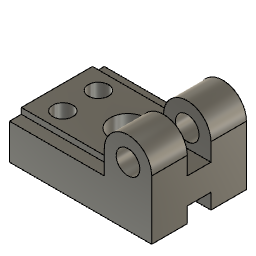
drawing_16 v1 (Autodesk Fusion 360 design; units mm, degrees)
Autodesk Fusion 360 part; units mm, degrees
sketch "Sketch1" plane through (0, 0, 0) normal (0, 0, 1) x (1, 0, 0)
  line L0 (0, 0) -> (-60, 0)
  line L1 (-60, 0) -> (60, 0)
  line L2 (-60, 0) -> (-60, 40)
  line L3 (60, 0) -> (60, -40)
  line L4 (-60, 40) -> (60, 40)
  line L5 (60, 40) -> (60, -40)
  line L6 (60, -40) -> (-60, -40)
  line L7 (-60, -40) -> (-60, 40)
  dimension "d1" = 60
  dimension "d2" = 120
  dimension "d3" = 40
  dimension "d4" = 40
  constraint coincident L0.start origin
  constraint horizontal L0
  constraint parallel L0 L1
  constraint perpendicular L0 L2
  constraint perpendicular L1 L3
  constraint horizontal L4
  constraint vertical L5
  constraint horizontal L6
  constraint vertical L7
  measures "d1" distance of L0.start L0.end
  measures "d2" distance of L0.end L1.end
  measures "d3" distance of L0.end L2.end
  measures "d4" distance of L1.end L3.end
extrude "Extrude1" add sketch "Sketch1" along normal blind 35
sketch "Sketch2" plane through (0, 0, 35) normal (0, 0, 1) x (-1, 0, 0)
  line L0 (60, 40) -> (-60, 40)
  line L1 (-60, 40) -> (-60, -40)
  line L2 (-60, -40) -> (60, -40)
  line L3 (60, -40) -> (60, 40)
  line L4 (-60, -40) -> (40, -40)
  line L5 (60, 0) -> (60, -15)
  line L6 (60, 0) -> (60, 15)
  circle A0 centre (40, -15) radius 8.5
  circle A1 centre (40, 15) radius 8.5
  dimension "d10" = 17
  dimension "d11" = 17
  constraint coincident L1.end L2.start
  constraint perpendicular L1 L4
  constraint midpoint L3 L5.start
  constraint parallel L3 L5
  constraint parallel L3 L6
  measures "d10" diameter of A0
  measures "d11" diameter of A1
extrude "Extrude2" cut sketch "Sketch2" against normal blind 70 contours A0 | A1
sketch "Sketch3" plane through (0, 0, 35) normal (0, 0, 1) x (-1, 0, 0)
  circle A0 centre (40, -15) radius 8.5
  circle A1 centre (40, 15) radius 8.5
  line L0 (60, 40) -> (-60, 40)
  line L1 (-60, 40) -> (-60, -40)
  line L2 (-60, -40) -> (60, -40)
  line L3 (60, -40) -> (60, 40)
  line L4 (-60, 40) -> (0, 40)
  circle A2 centre (0, 0) radius 9
  dimension "d14" = 60
  dimension "d15" = 18
  constraint coincident L0.end L1.start
  constraint perpendicular L1 L4
  constraint coincident A2.centre origin
  measures "d14" distance of L0.end L4.end
  measures "d15" diameter of A2
extrude "Extrude3" cut sketch "Sketch3" against normal blind 55 contours A2
sketch "Sketch4" plane through (0, 0, 35) normal (0, 0, 1) x (-1, 0, 0)
  circle A0 centre (0, 0) radius 9
  circle A1 centre (40, -15) radius 8.5
  circle A2 centre (40, 15) radius 8.5
  line L0 (60, 40) -> (-60, 40)
  line L1 (-60, 40) -> (-60, -40)
  line L2 (-60, -40) -> (60, -40)
  line L3 (60, -40) -> (60, 40)
  circle A3 centre (0, 0) radius 15
  dimension "d18" = 30
  constraint coincident A0.centre A3.centre
  measures "d18" diameter of A3
extrude "Extrude4" cut sketch "Sketch4" against normal blind 17 contours A3
sketch "Sketch5" plane through (0, 40, 0) normal (0, 1, 0) x (-1, 0, 0)
  line L0 (-60, 0) -> (60, 0)
  line L1 (60, 0) -> (60, 35)
  line L2 (60, 35) -> (-60, 35)
  line L3 (-60, 35) -> (-60, 0)
  line L4 (-60, 0) -> (-40, 0)
  line L5 (-60, 0) -> (-60, 50)
  line L6 (-20, 50) -> (-20, 0)
  arc A0 (-20, 50) -> (-60, 50) centre (-40, 50) ccw
  dimension "d21" = 20
  dimension "d22" = 50
  dimension "d23" = 40
  constraint coincident L0.start L3.end
  constraint perpendicular L3 L4
  constraint tangent L5 A0
  constraint coincident L0 L6.end
  constraint tangent L6 A0
  constraint perpendicular L0 L6
  measures "d21" distance of L0.start L4.end
  measures "d22" distance of L4.end A0.centre
  measures "d23" diameter of A0
extrude "Extrude5" add sketch "Sketch5" against normal blind 80 contours L0 L2 L3 L4 L5 L6 | L2 L5 L6 A0
sketch "Sketch6" plane through (0, 40, 0) normal (0, 1, 0) x (-1, 0, 0)
  line L0 (-60, 0) -> (60, 0)
  line L1 (60, 0) -> (60, 35)
  line L2 (60, 35) -> (-20, 35)
  line L3 (-20, 35) -> (-20, 50)
  arc A0 (-20, 50) -> (-60, 50) centre (-40, 50) ccw
  line L4 (-60, 50) -> (-60, 0)
  circle A1 centre (-40, 50) radius 10
  dimension "d26" = 20
  constraint concentric A0 A1
  measures "d26" diameter of A1
extrude "Extrude6" cut sketch "Sketch6" against normal blind 95 contours A1
sketch "Sketch7" plane through (0, 0, 35) normal (0, 0, 1) x (-1, 0, 0)
  line L0 (-20, 40) -> (-20, -40)
  line L1 (-20, -40) -> (60, -40)
  line L2 (60, -40) -> (60, 40)
  line L3 (60, 40) -> (-20, 40)
  circle A0 centre (0, 0) radius 15
  circle A1 centre (40, -15) radius 8.5
  circle A2 centre (40, 15) radius 8.5
  line L4 (60, 40) -> (60, 30) construction
  line L5 (60, -40) -> (60, -30) construction
  line L6 (60, -40) -> (-20, -40)
  line L7 (-20, -40) -> (-20, -30)
  line L8 (-20, -30) -> (60, -30)
  line L9 (60, -30) -> (60, -40)
  line L10 (60, 30) -> (-20, 30)
  line L11 (-20, 30) -> (-20, 40)
  line L12 (-20, 40) -> (60, 40)
  line L13 (60, 40) -> (60, 30)
  constraint coincident L2.end L3.start
  constraint perpendicular L3 L4
  constraint coincident L1.end L2.start
  constraint coincident L2 L5.end
  constraint perpendicular L1 L5
  constraint horizontal L6
  constraint vertical L7
  constraint horizontal L8
  constraint vertical L9
  constraint coincident L0 L7.end
  constraint horizontal L10
  constraint vertical L11
  constraint horizontal L12
  constraint vertical L13
  constraint coincident L0.start L3.end
extrude "Extrude7" cut sketch "Sketch7" against normal blind 5 contours L0 L2 L3 L10 L11 L12 L13 | L0 L1 L2 L6 L7 L8 L9
ref_plane "WorkPlane1" through (0, 0, 35) normal (0, 0, 1) x (1, 0, 0)
sketch "Sketch8" plane through (0, 0, 35) normal (0, 0, 1) x (1, 0, 0)
  line L0 (60, -40) -> (-60, -40)
  line L1 (-60, -40) -> (-60, 40)
  line L2 (-60, 40) -> (60, 40)
  line L3 (60, 40) -> (60, -40)
  circle A0 centre (-40, -15) radius 8.5
  circle A1 centre (-40, 15) radius 8.5
  circle A2 centre (0, 0) radius 9
  line L4 (60, 0) -> (30, 0) construction
  line L5 (30, 0) -> (20, 0) construction
  line L6 (20, 0) -> (20, 10) construction
  line L7 (20, 10) -> (20, -10)
  line L8 (20, -10) -> (67.6256, -10)
  line L9 (67.6256, -10) -> (67.6256, 10)
  line L10 (67.6256, 10) -> (20, 10)
  dimension "d33" = 30
  dimension "d34" = 10
  dimension "d35" = 20
  constraint horizontal L4
  constraint parallel L4 L5
  constraint perpendicular L5 L6
  constraint perpendicular L5 L7
  constraint perpendicular L3 L8
  constraint perpendicular L8 L9
  constraint perpendicular L7 L10
  measures "d33" distance of L4.start L4.end
  measures "d34" distance of L5.end L6.end
  measures "d35" distance of L6.end L7.end
extrude "Extrude8" cut sketch "Sketch8" along normal blind 90 contours L3 L7 L8 L10 | L3 L8 L9 L10
sketch "Sketch9" plane through (0, 0, 0) normal (0, 0, -1) x (1, 0, 0)
  line L0 (60, 40) -> (-60, 40)
  line L1 (-60, 40) -> (-60, -40)
  line L2 (-60, -40) -> (60, -40)
  line L3 (60, -40) -> (60, 40)
  circle A0 centre (-40, 15) radius 8.5
  circle A1 centre (-40, -15) radius 8.5
  circle A2 centre (0, 0) radius 9
  line L4 (60, 0) -> (20, 0) construction
  line L5 (60, 0) -> (30, 0) construction
  line L6 (30, -10) -> (73.1497, -10)
  arc A3 (73.1497, -10) -> (73.1497, 10) centre (73.1497, 0) ccw
  line L7 (73.1497, 10) -> (30, 10)
  arc A4 (30, 10) -> (30, -10) centre (30, 0) ccw
  line L8 (20, 0) -> (83.1497, 0) construction
  dimension "d38" = 40
  dimension "d39" = 30
  dimension "d40" = 20
  constraint midpoint L3 L4.start
  constraint perpendicular L3 L4
  constraint perpendicular L3 L5
  constraint tangent L6 A3
  constraint tangent A3 L7
  constraint parallel L6 L7
  constraint tangent L7 A4
  constraint tangent L6 A4
  constraint midpoint L4.end A4
  constraint midpoint A3 L8.end
  constraint perpendicular L3 L8
  measures "d38" distance of L4.start L4.end
  measures "d39" distance of L4.start L5.end
  measures "d40" diameter of A3
extrude "Extrude9" cut sketch "Sketch9" against normal blind 13 contours L3 L6 L7 A4
